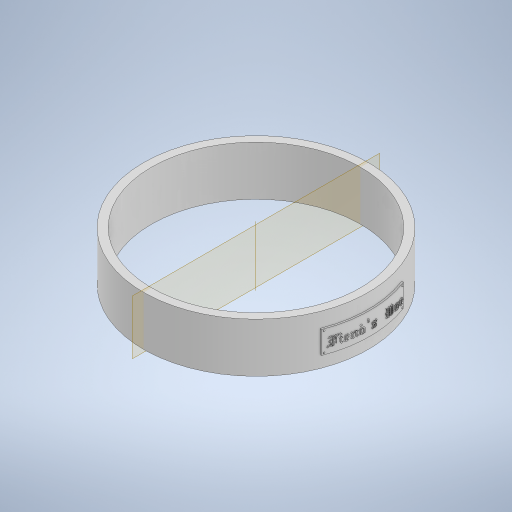
# Autodesk Inventor part: FiendsWoe
Saved by Autodesk Inventor 2023 (Build 270158000, 158)
## iProperties
Created: 2023-04-08
Part Number: FiendsWoe
Material: Generic
Document SubType Name: Modeling
Designer: dntpa
Density: 1 g/cm^3
Appearance: Default
Author: dntpa
## iProperties of the stored document CanisInvictoria_3DPrint.ipt
Created: 2023-04-08
Part Number: CanisInvictoria_3DPrint
Material: Generic
Document SubType Name: Modeling
Designer: dntpa
Density: 1 g/cm^3
Appearance: Default
Author: dntpa
Autodesk Inventor part; units mm, degrees
ref_plane "XZ Plane" through (0, 0, 0) normal (0, 1, 0) x (-1, 0, 0)
ref_plane "XY Plane" through (0, 0, 0) normal (0, 0, 1) x (1, 0, 0)
sketch "Sketch1" plane through (0, 0, 0) normal (0, 1, 0) x (-1, 0, 0)
  circle A0 centre (0, 0) radius 50
  circle A1 centre (0, 0) radius 46.5
  dimension "d0" = 100
  dimension "d1" = 93
  constraints: 2 centre point, 2 coincident
  measures "d0" diameter of A0
  measures "d1" diameter of A1
extrude "Extrusion1" add sketch "Sketch1" along normal blind 22
ref_plane "Work Plane1" through (60, 0, 0) normal (1, 0, 0) x (0, 1, 0)
sketch "Text" plane through (60, 0, 0) normal (1, 0, 0) x (0, 1, 0)
  line L0 (15.4535, 18.5) -> (15.4535, -18.5) construction
  line L1 (15.4535, -18.5) -> (5.4535, -18.5) construction
  line L2 (5.4535, -18.5) -> (5.4535, 18.5) construction
  line L3 (5.4535, 18.5) -> (15.4535, 18.5) construction
  line L4 (22, -50) -> (22, 50) projected
  line L5 (5.4535, 18.5) -> (15.4535, 18.5)
  line L6 (15.4535, 18.5) -> (15.4535, -18.5)
  line L7 (15.4535, -18.5) -> (5.4535, -18.5)
  line L8 (5.4535, -18.5) -> (5.4535, 18.5)
  line L9 (15.4535, 18.5) -> (15.4535, 0)
  line L10 (15.4535, 0) -> (15.4535, -18.5)
  circle A0 centre (14.7035, 17.75) radius 0.375
  line L11 (22, 0) -> (0, 0)
  line L12 (10.4535, 18.5) -> (10.4535, -18.5)
  circle A1 centre (14.7035, -17.75) radius 0.375
  circle A2 centre (6.2035, 17.75) radius 0.375
  circle A3 centre (6.2035, -17.75) radius 0.375
  line L13 (12.2028, 12.6745) -> (11.5968, 12.9739)
  line L14 (11.5968, 12.9739) -> (11.4057, 13.3562)
  line L15 (11.4057, 13.3562) -> (11.4057, 13.688)
  line L16 (11.4057, 13.688) -> (8.9133, 13.688)
  line L17 (8.9133, 13.688) -> (8.9133, 13.7674)
  line L18 (8.9133, 13.7674) -> (9.9593, 13.7674)
  line L19 (9.9593, 13.7674) -> (9.9593, 14.2326)
  line L20 (9.9593, 14.2326) -> (8.9025, 14.2326)
  line L21 (8.9025, 14.2326) -> (8.5202, 14.4202)
  spline S0 degree 2 poles (8.5202, 14.4202) (8.43, 14.6078) (8.329, 14.7989) knots 0 0 0 1 1 1
  line L22 (8.329, 14.7989) -> (8.329, 14.8061)
  line L23 (8.329, 14.8061) -> (8.1487, 15.1668)
  line L24 (8.1487, 15.1668) -> (8.1487, 15.5491)
  line L25 (8.1487, 15.5491) -> (8.329, 15.9098)
  line L26 (8.329, 15.9098) -> (8.329, 16.2561)
  spline S1 degree 2 poles (8.329, 16.2561) (8.2677, 16.4473) (8.1523, 16.7971) (8.1018, 16.9594) knots 0 0 0 1 2 2 2
  line L27 (8.1018, 16.9594) -> (8.4264, 16.6312)
  spline S2 degree 2 poles (8.4264, 16.6312) (8.448, 16.6096) (8.531, 16.5266) (8.5887, 16.4689) knots 0 0 0 1 2 2 2
  line L28 (8.5887, 16.4689) -> (8.7763, 16.0938)
  line L29 (8.7763, 16.0938) -> (8.7763, 15.7078)
  line L30 (8.7763, 15.7078) -> (8.412, 14.9865)
  line L31 (8.412, 14.9865) -> (8.412, 14.8314)
  line L32 (8.412, 14.8314) -> (8.5671, 14.6763)
  line L33 (8.5671, 14.6763) -> (11.2902, 14.6763)
  line L34 (11.2902, 14.6763) -> (11.485, 14.2976)
  spline S3 degree 2 poles (11.485, 14.2976) (11.5211, 14.2615) (11.6149, 14.1677) (11.669, 14.1136) knots 0 0 0 1 2 2 2
  line L35 (11.669, 14.1136) -> (12.0405, 13.7385)
  line L36 (12.0405, 13.7385) -> (11.8493, 13.3562)
  line L37 (11.8493, 13.3562) -> (11.8493, 13.0207)
  line L38 (11.8493, 13.0207) -> (12.2028, 12.6745)
  spline S4 degree 2 poles (9.6275, 15.1344) (9.5481, 15.1704) (9.3606, 15.2642) (9.2488, 15.3219) knots 0 0 0 1 2 2 2
  spline S5 degree 2 poles (9.2488, 15.3219) (9.1983, 15.3724) (9.0756, 15.4986) (8.9963, 15.578) knots 0 0 0 1 2 2 2
  line L39 (8.9963, 15.578) -> (9.9593, 15.578)
  line L40 (9.9593, 15.578) -> (9.9593, 15.8846)
  line L41 (9.9593, 15.8846) -> (9.7213, 16.1226)
  line L42 (9.7213, 16.1226) -> (10.1974, 16.1226)
  line L43 (10.1974, 16.1226) -> (10.403, 15.9134)
  line L44 (10.403, 15.9134) -> (10.403, 15.578)
  line L45 (10.403, 15.578) -> (10.5508, 15.578)
  spline S6 degree 2 poles (10.5508, 15.578) (10.6338, 15.5419) (10.8177, 15.4482) (10.9296, 15.3904) knots 0 0 0 1 2 2 2
  spline S7 degree 2 poles (10.9296, 15.3904) (10.9801, 15.3399) (11.1063, 15.2137) (11.182, 15.1344) knots 0 0 0 1 2 2 2
  line L46 (11.182, 15.1344) -> (9.6275, 15.1344)
  line L47 (10.403, 13.771) -> (11.4201, 13.771)
  line L48 (11.4201, 13.771) -> (11.5752, 14.0812)
  line L49 (11.5752, 14.0812) -> (11.4309, 14.2326)
  line L50 (11.4309, 14.2326) -> (10.403, 14.2326)
  line L51 (10.403, 14.2326) -> (10.403, 13.771)
  line L52 (12.1379, 14.4202) -> (11.586, 14.9793)
  line L53 (11.586, 14.9793) -> (11.586, 15.5491)
  line L54 (11.586, 15.5491) -> (11.7627, 15.899)
  line L55 (11.7627, 15.899) -> (11.4778, 16.4761)
  line L56 (11.4778, 16.4761) -> (12.0296, 15.9134)
  line L57 (12.0296, 15.9134) -> (12.0296, 15.3472)
  line L58 (12.0296, 15.3472) -> (11.8529, 14.9973)
  line L59 (11.8529, 14.9973) -> (12.1379, 14.4202)
  line L60 (8.5923, 11.2498) -> (8.1342, 11.7078)
  line L61 (8.1342, 11.7078) -> (8.5346, 12.1118)
  line L62 (8.5346, 12.1118) -> (10.1541, 12.1118)
  line L63 (10.1541, 12.1118) -> (10.3597, 12.5266)
  spline S8 degree 2 poles (10.3597, 12.5266) (10.403, 12.4364) (10.5112, 12.2236) (10.5761, 12.0974) knots 0 0 0 1 2 2 2
  spline S9 degree 2 poles (10.5761, 12.0974) (10.5941, 12.0757) (10.7781, 11.8882) knots 0 0 0 1 1 1
  spline S10 degree 2 poles (10.7781, 11.8882) (10.5941, 11.7042) (10.5761, 11.6826) knots 0 0 0 1 1 1
  spline S11 degree 2 poles (10.5761, 11.6826) (10.5725, 11.6754) (10.4679, 11.4626) (10.3597, 11.2534) knots 0 0 0 1 2 2 2
  line L64 (10.3597, 11.2534) -> (10.1541, 11.6682)
  line L65 (10.1541, 11.6682) -> (8.7474, 11.6682)
  line L66 (8.7474, 11.6682) -> (8.5923, 11.5131)
  line L67 (8.5923, 11.5131) -> (8.5923, 11.2498)
  line L68 (11.6149, 11.4554) -> (11.3984, 11.8918)
  line L69 (11.3984, 11.8918) -> (11.6149, 12.3246)
  line L70 (11.6149, 12.3246) -> (12.0441, 11.8918)
  line L71 (12.0441, 11.8918) -> (11.6149, 11.4554)
  line L72 (9.9882, 8.5374) -> (9.2488, 9.8251)
  line L73 (9.2488, 9.8251) -> (8.7582, 9.8251)
  line L74 (8.7582, 9.8251) -> (8.5923, 9.4932)
  line L75 (8.5923, 9.4932) -> (8.5923, 9.147)
  line L76 (8.5923, 9.147) -> (8.4228, 9.4896)
  spline S12 degree 2 poles (8.4228, 9.4896) (8.4012, 9.5257) (8.3579, 9.6123) (8.3326, 9.6592) knots 0 0 0 1 2 2 2
  spline S13 degree 2 poles (8.3326, 9.6592) (8.3218, 9.6736) (8.1342, 9.8647) knots 0 0 0 1 1 1
  spline S14 degree 2 poles (8.1342, 9.8647) (8.3146, 10.0487) (8.3507, 10.1064) knots 0 0 0 1 1 1
  spline S15 degree 2 poles (8.3507, 10.1064) (8.3543, 10.11) (8.43, 10.2651) (8.5094, 10.4166) knots 0 0 0 1 2 2 2
  line L77 (8.5094, 10.4166) -> (8.5094, 10.7665)
  line L78 (8.5094, 10.7665) -> (8.7582, 10.2687)
  line L79 (8.7582, 10.2687) -> (10.3921, 10.2687)
  line L80 (10.3921, 10.2687) -> (10.5833, 9.5185)
  spline S16 degree 2 poles (10.5833, 9.5185) (10.5905, 9.4968) (10.7745, 9.1326) knots 0 0 0 1 1 1
  line L81 (10.7745, 9.1326) -> (9.9882, 8.5374)
  line L82 (9.8114, 9.0063) -> (10.4895, 9.5149)
  line L83 (10.4895, 9.5149) -> (10.3344, 9.8251)
  line L84 (10.3344, 9.8251) -> (9.3461, 9.8251)
  line L85 (9.3461, 9.8251) -> (9.8114, 9.0063)
  line L86 (10.403, 5.3165) -> (10.1541, 5.8106)
  line L87 (10.1541, 5.8106) -> (8.7474, 5.8106)
  line L88 (8.7474, 5.8106) -> (8.5923, 5.6555)
  line L89 (8.5923, 5.6555) -> (8.5923, 5.3922)
  line L90 (8.5923, 5.3922) -> (8.1342, 5.8539)
  line L91 (8.1342, 5.8539) -> (8.5346, 6.2543)
  line L92 (8.5346, 6.2543) -> (10.1541, 6.2543)
  line L93 (10.1541, 6.2543) -> (10.3164, 6.5897)
  line L94 (10.3164, 6.5897) -> (10.3164, 6.752)
  line L95 (10.3164, 6.752) -> (10.1469, 7.2606)
  line L96 (10.1469, 7.2606) -> (8.7582, 7.2606)
  line L97 (8.7582, 7.2606) -> (8.5599, 6.8674)
  line L98 (8.5599, 6.8674) -> (8.1342, 7.3003)
  spline S17 degree 2 poles (8.1342, 7.3003) (8.3146, 7.4842) (8.3507, 7.5419) knots 0 0 0 1 1 1
  spline S18 degree 2 poles (8.3507, 7.5419) (8.3543, 7.5455) (8.43, 7.7006) (8.5094, 7.8521) knots 0 0 0 1 2 2 2
  line L99 (8.5094, 7.8521) -> (8.5094, 8.202)
  line L100 (8.5094, 8.202) -> (8.7582, 7.7042)
  line L101 (8.7582, 7.7042) -> (10.1649, 7.7042)
  line L102 (10.1649, 7.7042) -> (10.32, 7.8593)
  line L103 (10.32, 7.8593) -> (10.32, 8.1226)
  line L104 (10.32, 8.1226) -> (10.7781, 7.6646)
  line L105 (10.7781, 7.6646) -> (10.3777, 7.2606)
  line L106 (10.3777, 7.2606) -> (10.2334, 7.2606)
  spline S19 degree 2 poles (10.2334, 7.2606) (10.2551, 7.174) (10.338, 6.9324) (10.3957, 6.7737) knots 0 0 0 1 2 2 2
  line L107 (10.3957, 6.7737) -> (10.5148, 6.5392)
  spline S20 degree 2 poles (10.5148, 6.5392) (10.5292, 6.5068) (10.5797, 6.4202) knots 0 0 0 1 1 1
  spline S21 degree 2 poles (10.5797, 6.4202) (10.5905, 6.4058) (10.7781, 6.2146) knots 0 0 0 1 1 1
  spline S22 degree 2 poles (10.7781, 6.2146) (10.5977, 6.0343) (10.5581, 5.9693) knots 0 0 0 1 1 1
  spline S23 degree 2 poles (10.5581, 5.9693) (10.54, 5.9513) (10.403, 5.6628) knots 0 0 0 1 1 1
  line L108 (10.403, 5.6628) -> (10.403, 5.3165)
  line L109 (8.5094, 2.5212) -> (8.5094, 2.9216)
  spline S24 degree 2 poles (8.5094, 2.9216) (8.5058, 2.936) (8.4805, 3.0225) (8.4553, 3.0983) knots 0 0 0 1 2 2 2
  line L110 (8.4553, 3.0983) -> (8.3362, 3.4518)
  spline S25 degree 2 poles (8.3362, 3.4518) (8.3002, 3.5167) (8.2064, 3.7115) (8.1415, 3.8413) knots 0 0 0 1 2 2 2
  line L111 (8.1415, 3.8413) -> (8.3362, 4.0361)
  spline S26 degree 2 poles (8.3362, 4.0361) (8.3975, 4.1695) (8.5094, 4.3859) knots 0 0 0 1 1 1
  line L112 (8.5094, 4.3859) -> (8.5094, 4.9125)
  line L113 (8.5094, 4.9125) -> (8.7582, 4.4148)
  line L114 (8.7582, 4.4148) -> (10.3921, 4.4148)
  line L115 (10.3921, 4.4148) -> (10.4535, 4.2236)
  line L116 (10.4535, 4.2236) -> (10.5797, 3.8449)
  line L117 (10.5797, 3.8449) -> (10.7348, 3.5419)
  line L118 (10.7348, 3.5419) -> (11.6329, 4.44)
  line L119 (11.6329, 4.44) -> (12.0513, 3.8088)
  line L120 (12.0513, 3.8088) -> (11.467, 3.6105)
  line L121 (11.467, 3.6105) -> (10.3777, 2.5212)
  line L122 (10.3777, 2.5212) -> (8.5094, 2.5212)
  line L123 (8.5815, 2.9648) -> (10.1649, 2.9648)
  line L124 (10.1649, 2.9648) -> (10.6699, 3.4734)
  line L125 (10.6699, 3.4734) -> (10.338, 3.9711)
  line L126 (10.338, 3.9711) -> (8.7582, 3.9711)
  spline S27 degree 2 poles (8.7582, 3.9711) (8.7294, 3.9062) (8.6428, 3.7295) (8.5887, 3.6249) knots 0 0 0 1 2 2 2
  line L127 (8.5887, 3.6249) -> (8.4156, 3.459)
  line L128 (8.4156, 3.459) -> (8.5815, 2.9648)
  line L129 (11.9792, 0.6853) -> (11.5968, 0.8765)
  line L130 (11.5968, 0.8765) -> (11.4093, 1.248)
  line L131 (11.4093, 1.248) -> (11.4814, 1.2913)
  line L132 (11.4814, 1.2913) -> (11.6545, 0.9486)
  line L133 (11.6545, 0.9486) -> (11.9755, 0.9486)
  line L134 (11.9755, 0.9486) -> (12.3507, 1.3237)
  line L135 (12.3507, 1.3237) -> (12.8051, 0.8945)
  line L136 (12.8051, 0.8945) -> (12.3615, 0.6853)
  line L137 (12.3615, 0.6853) -> (11.9792, 0.6853)
  line L138 (10.9332, -2.7124) -> (10.5364, -2.5176)
  spline S28 degree 2 poles (10.5364, -2.5176) (10.4787, -2.4959) (10.338, -2.4166) knots 0 0 0 1 1 1
  line L139 (10.338, -2.4166) -> (9.9737, -2.1749)
  spline S29 degree 2 poles (9.9737, -2.1749) (9.9485, -2.1569) (9.8583, -2.0992) (9.7934, -2.0523) knots 0 0 0 1 2 2 2
  spline S30 degree 2 poles (9.7934, -2.0523) (9.7393, -1.9982) (9.5914, -1.8503) (9.5012, -1.7565) knots 0 0 0 1 2 2 2
  line L140 (9.5012, -1.7565) -> (9.5012, -2.211)
  line L141 (9.5012, -2.211) -> (9.3029, -2.6041)
  line L142 (9.3029, -2.6041) -> (8.5238, -2.6041)
  line L143 (8.5238, -2.6041) -> (8.3362, -2.0415)
  line L144 (8.3362, -2.0415) -> (8.3218, -2.0307)
  line L145 (8.3218, -2.0307) -> (8.329, -2.0234)
  line L146 (8.329, -2.0234) -> (8.1487, -1.6592)
  line L147 (8.1487, -1.6592) -> (8.3326, -1.2876)
  line L148 (8.3326, -1.2876) -> (8.3326, -0.9486)
  line L149 (8.3326, -0.9486) -> (8.1559, -0.5951)
  line L150 (8.1559, -0.5951) -> (8.1956, -0.5699)
  line L151 (8.1956, -0.5699) -> (8.2208, -0.5446)
  line L152 (8.2208, -0.5446) -> (8.4625, -0.725)
  line L153 (8.4625, -0.725) -> (8.9386, -1.0857)
  line L154 (8.9386, -1.0857) -> (9.4147, -1.5618)
  line L155 (9.4147, -1.5618) -> (9.4147, -1.1073)
  line L156 (9.4147, -1.1073) -> (9.6131, -0.7142)
  line L157 (9.6131, -0.7142) -> (10.3921, -0.7142)
  line L158 (10.3921, -0.7142) -> (10.4498, -0.9053)
  line L159 (10.4498, -0.9053) -> (10.5761, -1.284)
  line L160 (10.5761, -1.284) -> (10.7672, -1.6592)
  line L161 (10.7672, -1.6592) -> (10.5833, -2.0307)
  line L162 (10.5833, -2.0307) -> (10.5833, -2.3661)
  line L163 (10.5833, -2.3661) -> (10.9332, -2.7124)
  line L164 (8.5671, -2.1605) -> (9.2488, -2.1605)
  line L165 (9.2488, -2.1605) -> (9.4147, -1.8287)
  line L166 (9.4147, -1.8287) -> (9.4147, -1.6736)
  line L167 (9.4147, -1.6736) -> (9.2379, -1.5005)
  line L168 (9.2379, -1.5005) -> (8.8881, -1.147)
  spline S31 degree 2 poles (8.8881, -1.147) (8.8628, -1.1289) (8.7763, -1.064) (8.7113, -1.0171) knots 0 0 0 1 2 2 2
  line L169 (8.7113, -1.0171) -> (8.3615, -0.7502)
  line L170 (8.3615, -0.7502) -> (8.5923, -1.1073)
  line L171 (8.5923, -1.1073) -> (8.5923, -1.67)
  line L172 (8.5923, -1.67) -> (8.4228, -2.009)
  line L173 (8.4228, -2.009) -> (8.5671, -2.1605)
  line L174 (10.5112, -2.413) -> (10.5003, -2.3986)
  line L175 (10.5003, -2.3986) -> (10.5003, -2.3913)
  line L176 (10.5003, -2.3913) -> (10.32, -2.0307)
  line L177 (10.32, -2.0307) -> (10.32, -1.6483)
  line L178 (10.32, -1.6483) -> (10.4931, -1.3057)
  line L179 (10.4931, -1.3057) -> (10.3452, -1.1578)
  line L180 (10.3452, -1.1578) -> (9.6636, -1.1578)
  line L181 (9.6636, -1.1578) -> (9.5012, -1.4896)
  line L182 (9.5012, -1.4896) -> (9.5012, -1.6411)
  line L183 (9.5012, -1.6411) -> (9.8475, -1.9874)
  spline S32 degree 2 poles (9.8475, -1.9874) (9.8655, -2.0018) (9.9557, -2.0595) (10.0242, -2.1064) knots 0 0 0 1 2 2 2
  line L184 (10.0242, -2.1064) -> (10.3813, -2.3481)
  spline S33 degree 2 poles (10.3813, -2.3481) (10.3885, -2.3481) (10.4498, -2.3805) (10.5112, -2.413) knots 0 0 0 1 2 2 2
  line L185 (8.7005, -11.174) -> (8.513, -10.6114)
  line L186 (8.513, -10.6114) -> (8.1198, -10.2182)
  line L187 (8.1198, -10.2182) -> (8.5202, -10.0162)
  line L188 (8.5202, -10.0162) -> (8.6861, -9.6808)
  line L189 (8.6861, -9.6808) -> (8.513, -9.165)
  line L190 (8.513, -9.165) -> (8.1342, -8.7827)
  line L191 (8.1342, -8.7827) -> (8.3326, -8.5807)
  spline S34 degree 2 poles (8.3326, -8.5807) (8.3759, -8.4581) (8.4661, -8.1948) (8.5094, -8.0541) knots 0 0 0 1 2 2 2
  line L192 (8.5094, -8.0541) -> (8.5094, -7.3399)
  line L193 (8.5094, -7.3399) -> (8.7582, -7.8377)
  line L194 (8.7582, -7.8377) -> (9.9557, -7.8377)
  line L195 (9.9557, -7.8377) -> (9.9557, -7.5311)
  line L196 (9.9557, -7.5311) -> (9.7213, -7.2931)
  line L197 (9.7213, -7.2931) -> (10.1938, -7.2931)
  line L198 (10.1938, -7.2931) -> (10.403, -7.5023)
  line L199 (10.403, -7.5023) -> (10.403, -7.8377)
  line L200 (10.403, -7.8377) -> (11.2578, -7.8377)
  spline S35 degree 2 poles (11.2578, -7.8377) (11.384, -7.7944) (11.6437, -7.7078) (11.788, -7.661) knots 0 0 0 1 2 2 2
  line L201 (11.788, -7.661) -> (12.1379, -7.3039)
  line L202 (12.1379, -7.3039) -> (11.9395, -7.7042)
  spline S36 degree 2 poles (11.9395, -7.7042) (11.9287, -7.7331) (11.8782, -7.8305) (11.8421, -7.9026) knots 0 0 0 1 2 2 2
  line L203 (11.8421, -7.9026) -> (11.6545, -8.0938)
  line L204 (11.6545, -8.0938) -> (11.2758, -8.2813)
  line L205 (11.2758, -8.2813) -> (8.7727, -8.2813)
  line L206 (8.7727, -8.2813) -> (8.7727, -8.7394)
  line L207 (8.7727, -8.7394) -> (11.6473, -8.7394)
  line L208 (11.6473, -8.7394) -> (12.0405, -9.3309)
  line L209 (12.0405, -9.3309) -> (11.6401, -9.7277)
  line L210 (11.6401, -9.7277) -> (8.7727, -9.7277)
  line L211 (8.7727, -9.7277) -> (8.7727, -10.1858)
  line L212 (8.7727, -10.1858) -> (11.6473, -10.1858)
  line L213 (11.6473, -10.1858) -> (12.0405, -10.7737)
  line L214 (12.0405, -10.7737) -> (11.6401, -11.174)
  line L215 (11.6401, -11.174) -> (8.7005, -11.174)
  line L216 (8.751, -10.7304) -> (9.7754, -10.7304)
  line L217 (9.7754, -10.7304) -> (9.7754, -10.2723)
  line L218 (9.7754, -10.2723) -> (8.7582, -10.2723)
  line L219 (8.7582, -10.2723) -> (8.6031, -10.5789)
  line L220 (8.6031, -10.5789) -> (8.751, -10.7304)
  line L221 (8.751, -9.284) -> (9.7754, -9.284)
  line L222 (9.7754, -9.284) -> (9.7754, -8.826)
  line L223 (9.7754, -8.826) -> (8.7582, -8.826)
  line L224 (8.7582, -8.826) -> (8.6031, -9.1362)
  line L225 (8.6031, -9.1362) -> (8.751, -9.284)
  line L226 (10.5833, -9.284) -> (11.4309, -9.284)
  line L227 (11.4309, -9.284) -> (11.586, -9.1289)
  line L228 (11.586, -9.1289) -> (11.586, -8.826)
  line L229 (11.586, -8.826) -> (10.5833, -8.826)
  line L230 (10.5833, -8.826) -> (10.5833, -9.284)
  line L231 (10.5833, -10.7304) -> (11.4309, -10.7304)
  line L232 (11.4309, -10.7304) -> (11.586, -10.5753)
  line L233 (11.586, -10.5753) -> (11.586, -10.2723)
  line L234 (11.586, -10.2723) -> (10.5833, -10.2723)
  line L235 (10.5833, -10.2723) -> (10.5833, -10.7304)
  line L236 (9.8583, -9.284) -> (10.5003, -9.284)
  line L237 (10.5003, -9.284) -> (10.5003, -8.826)
  line L238 (10.5003, -8.826) -> (9.8583, -8.826)
  line L239 (9.8583, -8.826) -> (9.8583, -9.284)
  line L240 (9.8583, -10.7304) -> (10.5003, -10.7304)
  line L241 (10.5003, -10.7304) -> (10.5003, -10.2723)
  line L242 (10.5003, -10.2723) -> (9.8583, -10.2723)
  line L243 (9.8583, -10.2723) -> (9.8583, -10.7304)
  line L244 (10.403, -14.9576) -> (10.1577, -14.4635)
  line L245 (10.1577, -14.4635) -> (8.5094, -14.4635)
  line L246 (8.5094, -14.4635) -> (8.5094, -14.0631)
  spline S37 degree 2 poles (8.5094, -14.0631) (8.5058, -14.0487) (8.4805, -13.9621) (8.4553, -13.8864) knots 0 0 0 1 2 2 2
  line L247 (8.4553, -13.8864) -> (8.3362, -13.5329)
  spline S38 degree 2 poles (8.3362, -13.5329) (8.3002, -13.468) (8.2064, -13.2732) (8.1415, -13.1434) knots 0 0 0 1 2 2 2
  line L248 (8.1415, -13.1434) -> (8.3362, -12.9486)
  spline S39 degree 2 poles (8.3362, -12.9486) (8.3975, -12.8151) (8.5094, -12.5987) knots 0 0 0 1 1 1
  line L249 (8.5094, -12.5987) -> (8.5094, -12.0721)
  line L250 (8.5094, -12.0721) -> (8.7582, -12.5699)
  line L251 (8.7582, -12.5699) -> (10.403, -12.5699)
  line L252 (10.403, -12.5699) -> (10.403, -12.9702)
  spline S40 degree 2 poles (10.403, -12.9702) (10.4102, -12.9811) (10.4354, -13.0712) (10.4607, -13.1434) knots 0 0 0 1 2 2 2
  line L253 (10.4607, -13.1434) -> (10.5797, -13.5005)
  spline S41 degree 2 poles (10.5797, -13.5005) (10.6122, -13.569) (10.7095, -13.7601) (10.7745, -13.8864) knots 0 0 0 1 2 2 2
  spline S42 degree 2 poles (10.7745, -13.8864) (10.7276, -13.9369) (10.6302, -14.0343) (10.5797, -14.0848) knots 0 0 0 1 2 2 2
  spline S43 degree 2 poles (10.5797, -14.0848) (10.5725, -14.0956) (10.4859, -14.2651) (10.403, -14.431) knots 0 0 0 1 2 2 2
  line L254 (10.403, -14.431) -> (10.403, -14.9576)
  line L255 (8.5815, -14.0198) -> (10.1541, -14.0198)
  spline S44 degree 2 poles (10.1541, -14.0198) (10.1829, -13.9513) (10.2695, -13.7782) (10.3236, -13.67) knots 0 0 0 1 2 2 2
  spline S45 degree 2 poles (10.3236, -13.67) (10.3633, -13.6339) (10.4462, -13.5509) (10.4967, -13.5077) knots 0 0 0 1 2 2 2
  line L256 (10.4967, -13.5077) -> (10.3308, -13.0135)
  line L257 (10.3308, -13.0135) -> (8.7582, -13.0135)
  spline S46 degree 2 poles (8.7582, -13.0135) (8.7294, -13.0784) (8.6428, -13.2552) (8.5887, -13.3598) knots 0 0 0 1 2 2 2
  line L258 (8.5887, -13.3598) -> (8.4156, -13.5257)
  line L259 (8.4156, -13.5257) -> (8.5815, -14.0198)
  line L260 (9.9882, -17.5906) -> (9.2488, -16.303)
  line L261 (9.2488, -16.303) -> (8.7582, -16.303)
  line L262 (8.7582, -16.303) -> (8.5923, -16.6348)
  line L263 (8.5923, -16.6348) -> (8.5923, -16.9811)
  line L264 (8.5923, -16.9811) -> (8.4228, -16.6384)
  spline S47 degree 2 poles (8.4228, -16.6384) (8.4012, -16.6023) (8.3579, -16.5158) (8.3326, -16.4689) knots 0 0 0 1 2 2 2
  spline S48 degree 2 poles (8.3326, -16.4689) (8.3218, -16.4545) (8.1342, -16.2633) knots 0 0 0 1 1 1
  spline S49 degree 2 poles (8.1342, -16.2633) (8.3146, -16.0794) (8.3507, -16.0216) knots 0 0 0 1 1 1
  spline S50 degree 2 poles (8.3507, -16.0216) (8.3543, -16.018) (8.43, -15.8629) (8.5094, -15.7115) knots 0 0 0 1 2 2 2
  line L265 (8.5094, -15.7115) -> (8.5094, -15.3616)
  line L266 (8.5094, -15.3616) -> (8.7582, -15.8593)
  line L267 (8.7582, -15.8593) -> (10.3921, -15.8593)
  line L268 (10.3921, -15.8593) -> (10.5833, -16.6096)
  spline S51 degree 2 poles (10.5833, -16.6096) (10.5905, -16.6312) (10.7745, -16.9955) knots 0 0 0 1 1 1
  line L269 (10.7745, -16.9955) -> (9.9882, -17.5906)
  line L270 (9.8114, -17.1217) -> (10.4895, -16.6132)
  line L271 (10.4895, -16.6132) -> (10.3344, -16.303)
  line L272 (10.3344, -16.303) -> (9.3461, -16.303)
  line L273 (9.3461, -16.303) -> (9.8114, -17.1217)
  dimension "d6" = 11.5465
  dimension "d10" = 0
  dimension "d11" = 10
  dimension "d12" = 37
  dimension "d25" = 0.75
  dimension "d26" = 0.75
  dimension "d27" = 0.75
  constraints: 16 end point, 5 midpoint, 4 centre point, 3 symmetric about line, 2 collinear, 2 horizontal, 2 parallel, 1 perpendicular, 5 other
  measures "d6" distance from line of L4 L12.start
  measures "d10" vertical distance of L11.start point (15.453, 0)
  measures "d11" distance between parallel lines of L0 L2
  measures "d12" distance between parallel lines of L3 L1
  measures "d25" diameter of A0
  measures "d26" distance from line of L0 A0.centre
  measures "d27" distance from line of L3 A0.centre
sketch "NamePlate" plane through (60, 0, 0) normal (1, 0, 0) x (0, 1, 0)
  line L0 (15.4535, 18.5) -> (5.4535, 18.5)
  line L1 (5.4535, 18.5) -> (5.4535, -18.5)
  line L2 (5.4535, -18.5) -> (15.4535, -18.5)
  line L3 (15.4535, -18.5) -> (15.4535, 18.5)
  point P0 (0, 0)
  point P1 (15.4535, 18.5)
  point P2 (5.4535, -18.5)
  dimension "d19" = 0
  dimension "d20" = 0
  constraints: 8 end point, 2 parallel, 1 horizontal, 1 perpendicular
  measures "d19" distance from line of point (15.453, 18.5) L0
  measures "d20" distance from line of point (5.453, -18.5) L2
emboss "Emboss4" sketch "NamePlate" operation add depth 0.75 direction (1, 0, 0) wrap yes faces at (32.9673, 14.6667, 37.592)
emboss "Emboss5" sketch "Text" operation add depth 0.5 direction (1, 0, 0) wrap yes faces at (50.6671, 12.1201, -2.8993) contours L45 S6 S7 L46 L12 | L12 L46 S4 S5 L39 L40 L41 L42 L43 L44 L45 | L121 L122 L109 S24 L110 S25 L111 S26 L112 L113 L114 L115 L12 L125 L126 S27 L127 L128 L123 L124 | L12 L124 L125 L116 L117 L118 L119 L120 L121 | L159 L160 L161 L162 L163 L138 S28 L12 S33 L174 L175 L176 L178 L179 | L12 L179 L180 L181 L182 L183 S32 L184 S33 S28 L139 S29 S30 L140 L141 L142 L143 L144 L145 L146 L147 L148 L149 L150 L151 L152 L153 L154 L155 L156 L157 L158 L159 | L33 L34 S3 L35 L36 L37 L38 L13 L14 L15 L16 L12 L47 L48 L49 L50 | L12 L50 L51 L47 L16 L17 L18 L19 L20 L21 S0 L22 L23 L24 L25 L26 S1 L27 S2 L28 L29 L30 L31 L32 L33 | L269 L260 L261 L262 L263 L264 S47 S48 S49 S50 L265 L266 L267 L268 L12 L271 L272 L273 L270 | L12 L270 L271 L268 S51 L269 | L12 L176 L177 L178 | S23 L108 L86 L87 L88 L89 L90 L91 L92 L93 L94 L95 L96 L97 L98 S17 S18 L99 L100 L101 L102 L103 L104 L12 L105 L106 S19 L107 | L12 L107 S20 S21 S22 S23 | S8 S9 S10 S11 L12 | L12 S11 L64 L65 L66 L67 L60 L61 L62 L63 S8 | S43 L254 L244 L245 L246 S37 L247 S38 L248 S39 L249 L250 L251 L252 S40 L12 L256 L257 S46 L258 L259 L255 S44 S45 | L12 S45 L256 S40 L253 S41 S42 S43 | L12 L104 L105 | L200 S35 L201 L202 S36 L203 L204 L205 L12 | L12 L205 L206 L207 L238 L239 L236 L210 L211 L212 L242 L243 L240 L215 L185 L186 L187 L188 L189 L190 L191 S34 L192 L193 L194 L195 L196 L197 L198 L199 L200 | L80 S16 L81 L12 L82 L83 | L12 L83 L84 L85 L82 L81 L72 L73 L74 L75 L76 S12 S13 S14 S15 L77 L78 L79 L80 | L207 L208 L209 L210 L12 L236 L237 L238 | L12 L240 L241 L242 L212 L213 L214 L215 | L52 L53 L54 L55 L56 L57 L58 L59 | L68 L69 L70 L71 | L129 L130 L131 L132 L133 L134 L135 L136 L137
emboss "Emboss6" sketch "Text" operation add depth 0.4 direction (1, 0, 0) wrap yes faces at (49.1565, 14.3158, -12.6176) contours A0 | A1 | A2 | A3
fillet "Rivots" radius 0.35 4 edges at (48.0532, 14.3285, 17.5274) (48.0532, 5.8285, 17.5274) (48.0532, 14.3285, -17.5274) (48.0532, 5.8285, -17.5274)
pattern_circular "Circular Pattern1" count 2 over 360 about axis through (0, -10, 0) along (0, 1, 0) of "Emboss4"
pattern_circular "Circular Pattern2" count 2 over 360 about axis through (0, -10, 0) along (0, 1, 0) of "Emboss5"
pattern_circular "Circular Pattern3" count 2 over 360 about axis through (0, -10, 0) along (0, 1, 0) of "Emboss6"
body "Solid1"
